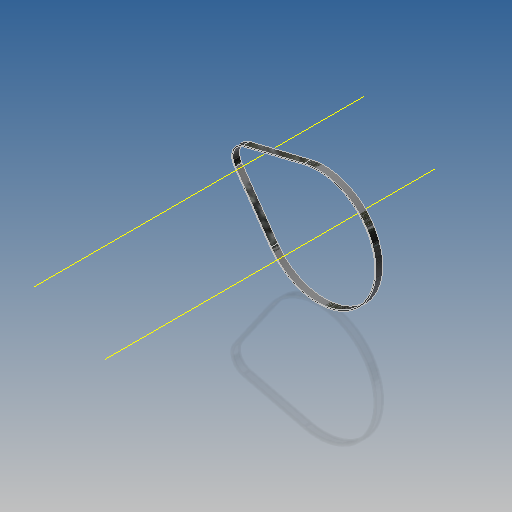
# Autodesk Inventor part: Correa síncrona
Saved by Autodesk Inventor 2017 (Build 210142000, 142)
## iProperties
Created: 2017-03-02
Part Number: Correa síncrona
Material: Rubber
Document SubType Name: Modeling
Designer: Leo
Density: 1 g/cm^3
Appearance: Rubber - Black - Version 1.1
CustomPartVersion: 1
Author: Leo
Autodesk Inventor part; units mm, degrees
sketch "Trayectoria de boceto" plane through (0, 0, 0) normal (0, 0, 1) x (1, 0, 0)
  arc A0 (-66.1313, 36.3002) -> (-73.5745, 16.6685) centre (-63.1158, 23.93) ccw
  arc A1 (-41.8348, -29.046) -> (-12.0619, 49.4806) centre (0, 0) ccw
  line L0 (-41.8348, -29.046) -> (-73.5745, 16.6685)
  line L1 (-66.1313, 36.3002) -> (-12.0619, 49.4806)
  constraints: 4 end point, 4 point on circle, 2 centre point
ref_plane "Plano de sección transversal" through (-73.5745, 16.6685, 0) normal (0.5703, -0.8214, 0) x (0, 0, 1)
ref_plane "Plano de trabajo2" through (-63.1158, 23.93, 0) normal (-1, 0, 0) x (0, 0, 1)
ref_plane "Plano de trabajo3" through (0, 0, 0) normal (-0.9816, -0.191, 0) x (0, 0, 1)
sketch "Sección transversal" plane through (-73.5745, 16.6685, 0) normal (0.5703, -0.8214, 0) x (0, 0, 1)
  line L0 (-3, 0.5) -> (3, 0.5)
  line L1 (3, 0.5) -> (3, -0.5)
  line L2 (3, -0.5) -> (-3, -0.5)
  line L3 (-3, -0.5) -> (-3, 0.5)
  line L4 (-3, 0) -> (3, 0) construction
  point P0 (0, 0)
  point P1 (0, 0)
  dimension "d0" = 6
  dimension "d4" = 0.5
  dimension "d5" = 0.5
  constraints: 10 end point, 3 midpoint, 2 parallel, 1 coincident, 1 horizontal, 1 perpendicular, 1 other
  measures "d0" distance between parallel lines of L1 L3
  measures "d4" distance between parallel lines of L2 L4
  measures "d5" distance between parallel lines of L4 L0
sweep "Correa" add profiles "Sección transversal" path "Trayectoria de boceto"
equation "\"d0\" = da_B"
equation "\"d4\" = da_a"
equation "\"d5\" = da_a2"
equation "\"da_B\" = 6"
equation "\"da_pb\" = 5"
equation "\"da_L\" = 357.25706"
equation "\"da_a\" = 0.5"
equation "\"da_S\" = 2.65"
equation "\"da_Beta\" = 20deg"
equation "\"da_Ht\" = 1.2"
equation "\"da_H\" = 2.2"
equation "\"da_a2\" = 0.5"
body "Solid1"
